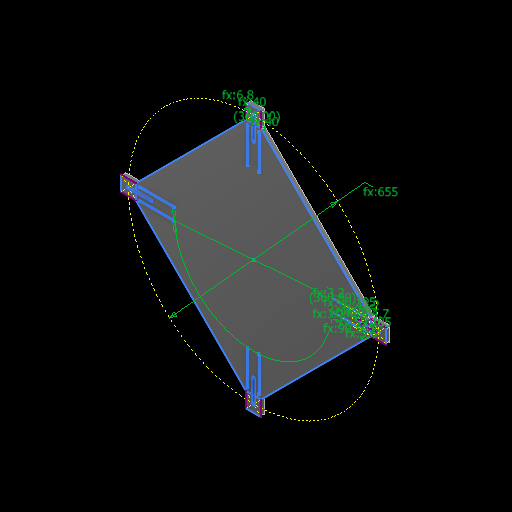
# Autodesk Inventor part: base_plate
Saved by Autodesk Inventor 2026.1 (Build 301233000, 233)
## iProperties
Created: 2025-09-14
Part Number: base_plate
Material: Aluminum 6061
Document SubType Name: Modeling
Designer: drago
Density: 2.7 g/cm^3
Appearance: Smooth - Black
Author: drago
Autodesk Inventor part; units mm, degrees
ref_plane "YZ Plane" through (0, 0, 0) normal (1, 0, 0) x (0, 1, 0)
ref_plane "XZ Plane" through (0, 0, 0) normal (0, 1, 0) x (-1, 0, 0)
ref_plane "XY Plane" through (0, 0, 0) normal (0, 0, 1) x (1, 0, 0)
sketch "Sketch2" plane through (0, 0, 0) normal (0, 0, 1) x (1, 0, 0)
  circle A0 centre (0, 0) radius 327.5 construction
  line L0 (-20, 307.5) -> (20, 307.5)
  line L1 (20, 307.5) -> (20, 347.5)
  line L2 (20, 347.5) -> (-20, 347.5)
  line L3 (-20, 347.5) -> (-20, 307.5)
  line L4 (-20, 307.5) -> (20, 347.5) construction
  line L5 (20, 307.5) -> (-20, 347.5) construction
  circle A1 centre (0, 327.5) radius 3.4
  circle A2 centre (-327.5, 0) radius 3.4
  line L6 (-347.5, 20) -> (-347.5, -20)
  line L7 (-347.5, -20) -> (-307.5, -20)
  line L8 (-307.5, -20) -> (-307.5, 20)
  line L9 (-307.5, 20) -> (-347.5, 20)
  line L10 (-307.5, 20) -> (-347.5, -20) construction
  line L11 (-307.5, -20) -> (-347.5, 20) construction
  circle A3 centre (0, -327.5) radius 3.4
  line L12 (-20, -347.5) -> (20, -347.5)
  line L13 (20, -347.5) -> (20, -307.5)
  line L14 (20, -307.5) -> (-20, -307.5)
  line L15 (-20, -307.5) -> (-20, -347.5)
  line L16 (-20, -307.5) -> (20, -347.5) construction
  line L17 (20, -307.5) -> (-20, -347.5) construction
  circle A4 centre (327.5, 0) radius 3.4
  line L18 (347.5, -20) -> (347.5, 20)
  line L19 (347.5, 20) -> (307.5, 20)
  line L20 (307.5, 20) -> (307.5, -20)
  line L21 (307.5, -20) -> (347.5, -20)
  line L22 (307.5, -20) -> (347.5, 20) construction
  line L23 (307.5, 20) -> (347.5, -20) construction
  line L24 (-20, 307.5) -> (-307.5, 20)
  line L25 (20, 307.5) -> (307.5, 20)
  line L26 (307.5, -20) -> (20, -307.5)
  line L27 (-20, -307.5) -> (-307.5, -20)
  line L28 (260.6, -21.1) -> (302.8, -21.1) construction
  line L29 (302.8, -21.1) -> (302.8, 21.1) construction
  line L30 (302.8, 21.1) -> (260.6, 21.1) construction
  line L31 (260.6, 21.1) -> (260.6, -21.1) construction
  line L32 (260.6, -21.1) -> (302.8, 21.1) construction
  line L33 (302.8, -21.1) -> (260.6, 21.1) construction
  line L34 (297.2, 15.5) -> (207.0955, 15.5) construction
  line L35 (297.2, 17.1) -> (207.0955, 17.1)
  line L36 (207.0955, 13.9) -> (297.2, 13.9)
  arc A5 (297.2, 13.9) -> (297.2, 17.1) centre (297.2, 15.5) ccw
  arc A6 (207.0955, 17.1) -> (207.0955, 13.9) centre (207.0955, 15.5) ccw
  line L37 (297.2, -15.5) -> (207.0955, -15.5) construction
  line L38 (297.2, -13.9) -> (207.0955, -13.9)
  line L39 (207.0955, -17.1) -> (297.2, -17.1)
  arc A7 (297.2, -17.1) -> (297.2, -13.9) centre (297.2, -15.5) ccw
  arc A8 (207.0955, -13.9) -> (207.0955, -17.1) centre (207.0955, -15.5) ccw
  line L40 (327.5, 0) -> (268.3955, 0) construction
  line L41 (327.5, 3.4) -> (268.3955, 3.4)
  line L42 (268.3955, -3.4) -> (327.5, -3.4)
  arc A9 (327.5, -3.4) -> (327.5, 3.4) centre (327.5, 0) ccw
  arc A10 (268.3955, 3.4) -> (268.3955, -3.4) centre (268.3955, 0) ccw
  arc A11 (-17.1, 207.0955) -> (-13.9, 207.0955) centre (-15.5, 207.0955) ccw
  line L43 (-17.1, 297.2) -> (-17.1, 207.0955)
  line L44 (-13.9, 207.0955) -> (-13.9, 297.2)
  arc A12 (-13.9, 297.2) -> (-17.1, 297.2) centre (-15.5, 297.2) ccw
  arc A13 (17.1, 297.2) -> (13.9, 297.2) centre (15.5, 297.2) ccw
  line L45 (13.9, 297.2) -> (13.9, 207.0955)
  line L46 (17.1, 207.0955) -> (17.1, 297.2)
  arc A14 (13.9, 207.0955) -> (17.1, 207.0955) centre (15.5, 207.0955) ccw
  line L47 (-3.4, 327.5) -> (-3.4, 268.3955)
  arc A15 (-3.4, 268.3955) -> (3.4, 268.3955) centre (0, 268.3955) ccw
  line L48 (3.4, 268.3955) -> (3.4, 327.5)
  circle A16 centre (0, 327.5) radius 3.4
  arc A17 (-207.0955, -17.1) -> (-207.0955, -13.9) centre (-207.0955, -15.5) ccw
  line L49 (-297.2, -17.1) -> (-207.0955, -17.1)
  line L50 (-207.0955, -13.9) -> (-297.2, -13.9)
  arc A18 (-297.2, -13.9) -> (-297.2, -17.1) centre (-297.2, -15.5) ccw
  arc A19 (-297.2, 17.1) -> (-297.2, 13.9) centre (-297.2, 15.5) ccw
  line L51 (-297.2, 13.9) -> (-207.0955, 13.9)
  line L52 (-207.0955, 17.1) -> (-297.2, 17.1)
  arc A20 (-207.0955, 13.9) -> (-207.0955, 17.1) centre (-207.0955, 15.5) ccw
  line L53 (-327.5, -3.4) -> (-268.3955, -3.4)
  arc A21 (-268.3955, -3.4) -> (-268.3955, 3.4) centre (-268.3955, 0) ccw
  line L54 (-268.3955, 3.4) -> (-327.5, 3.4)
  circle A22 centre (-327.5, 0) radius 3.4
  arc A23 (17.1, -207.0955) -> (13.9, -207.0955) centre (15.5, -207.0955) ccw
  line L55 (17.1, -297.2) -> (17.1, -207.0955)
  line L56 (13.9, -207.0955) -> (13.9, -297.2)
  arc A24 (13.9, -297.2) -> (17.1, -297.2) centre (15.5, -297.2) ccw
  arc A25 (-17.1, -297.2) -> (-13.9, -297.2) centre (-15.5, -297.2) ccw
  line L57 (-13.9, -297.2) -> (-13.9, -207.0955)
  line L58 (-17.1, -207.0955) -> (-17.1, -297.2)
  arc A26 (-13.9, -207.0955) -> (-17.1, -207.0955) centre (-15.5, -207.0955) ccw
  line L59 (3.4, -327.5) -> (3.4, -268.3955)
  arc A27 (3.4, -268.3955) -> (-3.4, -268.3955) centre (0, -268.3955) ccw
  line L60 (-3.4, -268.3955) -> (-3.4, -327.5)
  circle A28 centre (0, -327.5) radius 3.4
  point P0 (281.7, 0)
  point P1 (252.1478, 15.5)
  point P2 (252.1478, -15.5)
  point P3 (297.9478, 0)
  point P4 (3.4, -327.5)
  point P5 (3.4, 327.5)
  dimension "d26" = 655
  dimension "d28" = 40
  dimension "d29" = 40
  dimension "d30" = 6.8
  dimension "d33" = 360
  dimension "d110" = 42.2
  dimension "d112" = 4.7
  dimension "d113" = 42.2
  dimension "d114" = 3.2
  dimension "d115" = 90.1045
  dimension "d116" = 5.6
  dimension "d117" = 3.2
  dimension "d118" = 5.6
  dimension "d119" = 90.1045
  dimension "d122" = 59.1045
  dimension "d123" = 6.8
  dimension "d130" = 360
  constraints: 128 end point, 42 point on circle, 28 centre point, 12 tangent, 7 midpoint, 7 parallel, 5 horizontal, 4 coincident, 4 perpendicular, 2 point on line, 1 collinear, 1 vertical alignment, 176 other
  measures "d28" distance of L2.end L1.end
  measures "d29" distance of L1.end L0.end
  measures "d30" diameter of A1
  measures "d110" distance of L30.end L29.end
  measures "d112" distance between parallel lines of L20 L29
  measures "d113" distance between parallel lines of L28 L30
  measures "d114" diameter of A6
  measures "d115" distance of L34.start L34.end
  measures "d116" distance between parallel lines of L30 L34
  measures "d117" diameter of A8
  measures "d118" distance between parallel lines of L28 L37
  measures "d119" distance of L37.start L37.end
  measures "d122" distance of L40.start L40.end
  measures "d123" diameter of A10
extrude "Extrusion3" add sketch "Sketch2" against normal blind 10 contours L3 L2 L1 L0 L48 A1 L47 | L0 L47 A15 L48 L25 L20 L41 A10 L42 L26 L14 L59 A27 L60 L27 L8 L53 A21 L54 L24 | L47 A1 L48 L0 | L0 L48 A15 L47 | L8 L54 A2 L53 L7 L6 L9 | A1 | L54 A21 L53 L8 | L8 L53 A2 L54 | A2 | L19 L18 L21 L20 L42 A4 L41 | L41 A4 L42 L20 | L20 L42 A10 L41 | L14 L60 A3 L59 L13 L12 L15 | A4 | L60 A27 L59 L14 | L14 L59 A3 L60 | A3 | A5 L36 A6 L35 | A7 L39 A8 L38 | L43 A12 L44 A11 | L46 A14 L45 A13 | L49 A18 L50 A17 | L52 A20 L51 A19 | L55 A24 L56 A23 | L58 A26 L57 A25
fillet "Fillet5" radius 4 16 edges at (-307.5, 20, -5) (-347.5, 20, -5) (-347.5, -20, -5) (-20, -347.5, -5) (20, -347.5, -5) (-20, -307.5, -5) (-20, 347.5, -5) (307.5, -20, -5) (347.5, -20, -5) (347.5, 20, -5) (20, 307.5, -5) (20, 347.5, -5) (307.5, 20, -5) (-20, 307.5, -5) (-307.5, -20, -5) (20, -307.5, -5)
extrude "Extrusion8" cut sketch "Sketch2" against normal blind 10 contours L47 A1 L48 L0 | L0 L48 A15 L47 | A1 | L54 A21 L53 L8 | L8 L53 A2 L54 | A2 | L41 A4 L42 L20 | L20 L42 A10 L41 | A4 | L60 A27 L59 L14 | L14 L59 A3 L60 | A3 | A5 L36 A6 L35 | A7 L39 A8 L38 | L43 A12 L44 A11 | L46 A14 L45 A13 | L49 A18 L50 A17 | L52 A20 L51 A19 | L55 A24 L56 A23 | L58 A26 L57 A25
equation "\"d26\" = ring_outer_diam + bar_width"
equation "\"d28\" = bar_width"
equation "\"d29\" = bar_width"
equation "\"d30\" = bar_hole_diam"
equation "\"d35\" = base_plate_thick"
equation "\"ring_inner_diam\" = 565"
equation "\"bar_width\" = 40"
equation "\"bar_hole_diam\" = 6.8"
equation "\"ring_outer_diam\" = 615"
equation "\"base_plate_thick\" = 10"
equation "\"motor_width\" = 42.2"
equation "\"dist_motor_bar\" = 4.7"
equation "\"motor_slot_diam\" = 3.2"
equation "\"motor_slot_edge_dist\" = 5.6"
equation "\"motor_slot_length\" = 90.1045"
equation "\"bar_slot_diam\" = 6.8"
equation "\"bar_slot_length\" = 59.1045"
equation "\"dist_motor_holes\" = 31"
body "Solid2"
